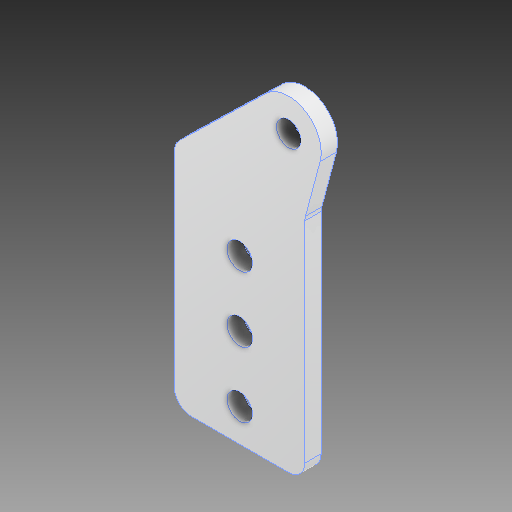
# Autodesk Inventor part: Top Bearing Plate (R4 - 0.25in Between Stages)
Saved by Autodesk Inventor 2022 (Build 260153000, 153)
## iProperties
Created: 2020-09-04
Part Number: Top Bearing Plate (R4 - 0.25in Between Stages)
Material: Aluminum 6061
Document SubType Name: Modeling
Density: 2.7 g/cm^3
Appearance: Aluminum - Flat
Mass: 10.4225 g
Surface Area: 31.0908 cm^2
Volume: 3.86019 cm^3
Autodesk Inventor part; units mm, degrees
ref_plane "YZ Plane" through (0, 0, 0) normal (1, 0, 0) x (0, 1, 0)
ref_plane "XZ Plane" through (0, 0, 0) normal (0, 1, 0) x (-1, 0, 0)
ref_plane "XY Plane" through (0, 0, 0) normal (0, 0, 1) x (1, 0, 0)
sketch "Sketch1" plane through (0, 0, 0) normal (0, 0, 1) x (1, 0, 0)
  arc A0 (6.1342, -1.6415) -> (-4.4197, 4.5595) centre (0, 0) ccw
  circle A1 centre (0, 0) radius 9.525 construction
  line L0 (3.175, -12.7) -> (-22.225, -12.7)
  line L1 (-22.225, -12.7) -> (-22.225, -63.5)
  line L2 (-22.225, -63.5) -> (3.175, -63.5)
  line L3 (3.175, -63.5) -> (3.175, -12.7)
  line L4 (3.175, -12.7) -> (-22.225, -63.5) construction
  line L5 (-22.225, -12.7) -> (3.175, -63.5) construction
  line L6 (9.525, 7.0623) -> (9.525, -12.9681) construction
  circle A2 centre (-9.525, -25.4) radius 2.4892
  circle A3 centre (-9.525, -38.1) radius 2.4892
  circle A4 centre (-9.525, -50.8) radius 2.4892
  circle A5 centre (0, 0) radius 2.3813
  line L7 (3.175, -12.7) -> (6.1342, -1.6415)
  line L8 (-4.4197, 4.5595) -> (-22.225, -12.7)
  line L9 (3.175, -63.5) -> (-22.225, -63.5)
  line L10 (-22.225, -63.5) -> (-22.225, -57.15)
  line L11 (-22.225, -57.15) -> (3.175, -57.15)
  line L12 (3.175, -57.15) -> (3.175, -63.5)
  line L13 (-22.225, -63.5) -> (-13.843, -63.5)
  line L14 (-13.843, -63.5) -> (-13.843, -44.45)
  line L15 (-13.843, -44.45) -> (-22.225, -44.45)
  line L16 (-22.225, -44.45) -> (-22.225, -63.5)
  point P0 (-13.843, -57.15)
  point P1 (3.175, -57.15)
  dimension "d0" = 12.7
  dimension "d1" = 19.05
  dimension "d2" = 25.4
  dimension "d4" = 6.35
  dimension "d5" = 4.9784
  dimension "d8" = 12.7
  dimension "d13" = 4.7625
  dimension "d17" = 3.175
  dimension "d18" = 12.7
  dimension "d19" = 6.35
  dimension "d20" = 8.382
  dimension "d21" = 19.05
  constraints: 34 end point, 6 centre point, 6 parallel, 4 coincident, 3 horizontal, 3 perpendicular, 3 tangent, 2 midpoint, 2 point on circle, 2 vertical, 1 point on line, 4 other
  measures "d0" diameter of A0
  measures "d1" diameter of A1
  measures "d2" distance between parallel lines of L3 L1
  measures "d4" distance between parallel lines of L3 L6
  measures "d5" diameter of A2
  measures "d8" distance of A2.centre A3.centre
  measures "d13" diameter of A5
  measures "d17" distance edge to line of A1 L0
  measures "d18" distance from line of L0 A2.centre
  measures "d19" distance between parallel lines of L9 L11
  measures "d20" distance of L15.end L14.end
  measures "d21" distance between parallel lines of L9 L15
extrude "Extrusion1" add sketch "Sketch1" along normal blind 3.175 contours L7 L0 L8 A0 | L3 L11 L14 L15 L1 L0 | L15 L14 L11 L1
fillet "Fillet1" radius 3.175 4 edges at (3.175, -12.7, 1.5875) (-22.225, -12.7, 1.5875) (3.175, -57.15, 1.5875) (-22.225, -57.15, 1.5875)
body "Solid1"
